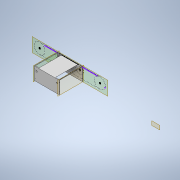
# Autodesk Inventor part: Podstawacz2
Saved by Autodesk Inventor 2022 (Build 260153000, 153)
## iProperties
Created: 2023-05-02
Part Number: Podstawacz2
Material: Ogólny
Document SubType Name: Modeling
Designer: nosal
Density: 1 g/cm^3
Appearance: Domyślna
Author: nosal
Autodesk Inventor part; units mm, degrees
sketch "Szkic1" plane through (0, 0, 0) normal (0, 0, 1) x (1, 0, 0)
  arc A0 (0, 35) -> (0, -35) centre (0, 0) ccw construction
  line L0 (0, 35) -> (390, 35) construction
  line L1 (0, -35) -> (390, -35) construction
  arc A1 (390, -35) -> (390, 35) centre (390, 0) ccw construction
  circle A2 centre (0, 0) radius 4.5
  circle A3 centre (390, 0) radius 4.5
  line L2 (130, 35) -> (130, 10) construction
  line L3 (260, 35) -> (260, 10) construction
  circle A4 centre (130, 10) radius 25 construction
  circle A5 centre (260, 10) radius 25 construction
  circle A6 centre (130, 10) radius 4.5
  circle A7 centre (260, 10) radius 4.5
  circle A8 centre (0, 0) radius 35 construction
  circle A9 centre (390, 0) radius 35 construction
  line L4 (117.8756, 33) -> (31.8551, 33)
  line L5 (375.6125, 33) -> (272.1244, 33)
  line L6 (247.8756, 33) -> (142.1244, 33)
  line L7 (31.8551, 31) -> (114.6703, 31)
  line L8 (145.3297, 31) -> (244.6703, 31)
  line L9 (275.3297, 31) -> (371.697, 31)
  arc A10 (375.6125, 33) -> (371.697, 31) centre (390, 0) ccw
  arc A11 (117.8756, 33) -> (114.6703, 31) centre (130, 10) ccw
  arc A12 (145.3297, 31) -> (142.1244, 33) centre (130, 10) ccw
  arc A13 (247.8756, 33) -> (244.6703, 31) centre (260, 10) ccw
  arc A14 (275.3297, 31) -> (272.1244, 33) centre (260, 10) ccw
  line L10 (31.8551, 14.5) -> (31.8551, 35) construction
  line L11 (31.8551, 33) -> (31.8551, 31)
  line L12 (260, 10) -> (260, 0)
  line L13 (130, 10) -> (130, 0)
  point P0 (423.5971, -9.8098)
  dimension "d94" = 50
  dimension "d0" = 70
  dimension "d1" = 390
  dimension "d2" = 390
  dimension "d3" = 70
  dimension "d4" = 9
  dimension "d5" = 9
  dimension "d10" = 25
  dimension "d11" = 25
  dimension "d12" = 9
  dimension "d13" = 9
  dimension "d14" = 130
  dimension "d15" = 260
  dimension "d24" = 2
  dimension "d25" = 2
  dimension "d26" = 2
  dimension "d27" = 1
  dimension "d95" = 2
  constraints: 28 end point, 17 point on circle, 13 centre point, 9 coincident, 6 point on line, 2 horizontal, 2 perpendicular, 2 tangent, 2 vertical, 2 vertical alignment, 1 concentric, 4 other
  measures "d0" diameter of A0
  measures "d1" distance of L0.start L0.end
  measures "d2" distance of L1.start L1.end
  measures "d3" diameter of A1
  measures "d4" diameter of A2
  measures "d5" diameter of A3
  measures "d10" distance of L2.start L2.end
  measures "d11" distance of L3.start L3.end
  measures "d12" diameter of A6
  measures "d13" diameter of A7
  measures "d14" distance between parallel lines of L3 L2
  measures "d15" distance from line of point (0, 0) L3
  measures "d24" distance between parallel lines of L4 L7
  measures "d25" distance between parallel lines of L6 L8
  measures "d26" distance between parallel lines of L5 L9
  measures "d27" radial gap between concentric circles of A9 A10
  measures "d95" distance between parallel lines of L0 L6
extrude "Wyciągnięcie proste1" add sketch "Szkic1" along normal blind 145 contours A11 L7 L11 L4 | A10 L9 A14 L5 | A13 L8 A12 L6
ref_plane "Płaszczyzna konstrukcyjna1" through (117.8756, 33, 145) normal (0, 0, 1) x (-1, 0, 0)
sketch "Szkic3" plane through (117.8756, 33, 145) normal (0, 0, 1) x (-1, 0, 0)
  circle A0 centre (117.8756, 33) radius 4.5 projected
  arc A1 (133.7659, 28.5) -> (133.7659, 37.5) centre (133.7659, 33) ccw
  arc A2 (98.6659, 37.5) -> (98.6659, 28.5) centre (98.6659, 33) ccw
  line L0 (133.7659, 28.5) -> (98.6659, 28.5)
  line L1 (98.6659, 37.5) -> (133.7659, 37.5)
  line L2 (98.6659, 18.5) -> (133.7659, 18.5)
  arc A3 (133.7659, 18.5) -> (133.7659, 47.5) centre (133.7659, 33) ccw
  line L3 (133.7659, 47.5) -> (98.6659, 47.5)
  line L4 (86.0205, 18.5) -> (86.0205, -2) construction
  line L5 (98.6659, 18.5) -> (86.0205, 18.5)
  line L6 (98.6659, 47.5) -> (86.0205, 47.5)
  line L7 (86.0205, 0) -> (86.0205, 2) projected
  line L8 (86.0205, 18.5) -> (86.0205, 0)
  line L9 (98.6659, 47.5) -> (98.6659, 81.8113)
  line L10 (98.6659, 81.8113) -> (-234.1244, 81.8113)
  line L11 (-157.4541, 2) -> (-253.8214, 2) projected
  line L12 (86.0205, 0) -> (86.0205, 2)
  line L13 (-257.7369, 0) -> (-154.2487, 0) projected
  line L14 (86.0205, 0) -> (-238.0399, 0)
  circle A4 centre (-272.1244, 33) radius 35 construction
  line L15 (-234.1244, 2) -> (-234.1244, 18.5)
  line L16 (-234.1244, 2) -> (-238.0399, 0)
  line L17 (-246.7694, 47.5) -> (-246.7694, 81.8113)
  line L18 (-246.7694, 81.8113) -> (-234.1244, 81.8113)
  line L19 (-303.9795, 47.5) -> (-409.6259, 47.5) construction
  line L20 (-234.1244, 47.5) -> (-246.7694, 47.5)
  line L21 (-234.1244, 18.5) -> (-281.8694, 18.5)
  line L22 (-246.7694, 47.5) -> (-281.8694, 47.5)
  arc A5 (-281.8694, 47.5) -> (-281.8694, 18.5) centre (-281.8694, 33) ccw
  point P0 (-238.0399, 0)
  dimension "d33" = 9
  dimension "d34" = 9
  dimension "d35" = 10
  dimension "d36" = 47.7454
  dimension "d37" = 12.6455
  dimension "d38" = 12.6455
  dimension "d39" = 12.6455
  dimension "d40" = 0
  dimension "d64" = 47.745
  dimension "d93" = 16.5
  constraints: 38 end point, 8 point on circle, 5 horizontal, 4 centre point, 3 parallel, 3 tangent, 3 vertical, 2 collinear, 2 perpendicular, 2 point on line, 4 other
  measures "d33" diameter of A1
  measures "d34" diameter of A2
  measures "d35" distance between parallel lines of L0 L2
  measures "d36" distance from line of L3.start L4
  measures "d37" distance from line of L3.end L4
  measures "d38" distance from line of L1.start L4
  measures "d39" distance from line of L2.start L4
  measures "d40" distance from line of L6.end L4
  measures "d64" distance of L15.end L21.end
  measures "d93" distance of L15.start L15.end
extrude "Wyciągnięcie proste2" add sketch "Szkic3" along normal blind 4
ref_plane "Płaszczyzna konstrukcyjna4" through (117.8756, 33, 72.5) normal (0, 0, -1) x (-1, 0, 0)
mirror "Odbij2" about plane through (117.8756, 33, 72.5) normal (0, 0, -1) of "Wyciągnięcie proste2"
extrude "Wyciągnięcie proste4" cut sketch "Szkic1" along normal mid plane 10000 contours A6 | A7
sketch "Szkic8" plane through (0, 0, 145) normal (0, 0, 1) x (1, 0, 0)
  line L0 (352, 31) -> (371.697, 31) projected
  line L1 (352, 31) -> (355.9155, 33) projected
  line L2 (352, 31) -> (355.9155, 33)
  line L3 (375.6125, 33) -> (355.9155, 33) projected
  line L4 (355.9155, 33) -> (375.6125, 33)
  arc A0 (375.6125, 33) -> (371.697, 31) centre (390, 0) ccw projected
  line L5 (375.6125, 33) -> (371.697, 31)
  line L6 (352, 14.5) -> (352, 31) projected
  line L7 (371.697, 31) -> (352, 31)
  point P0 (0, 0)
  point P1 (352, -48.8113)
  constraints: 8 end point, 3 equal length, 1 perpendicular
ref_plane "Płaszczyzna konstrukcyjna6" through (0, 0, 72.5) normal (0, 0, 1) x (1, 0, 0)
extrude "Wyciągnięcie proste5" cut sketch "Szkic8" along normal mid plane 1000 contours L1 L3 A0 L0
ref_plane "Płaszczyzna konstrukcyjna9" through (117.8756, 33, 149) normal (0, 0, 1) x (1, 0, 0)
sketch "Szkic12" plane through (117.8756, 33, 149) normal (0, 0, 1) x (1, 0, 0)
  line L0 (281.8694, -18.5) -> (234.1244, -18.5) projected
  arc A0 (281.8694, -47.5) -> (281.8694, -18.5) centre (281.8694, -33) ccw projected
  line L1 (246.7694, -47.5) -> (281.8694, -47.5) projected
  line L2 (246.7694, -81.8113) -> (246.7694, -47.5) projected
  line L3 (234.1244, -2) -> (234.1244, -81.8113) projected
  line L4 (-98.6659, -81.8113) -> (246.7694, -81.8113) projected
  point P0 (-117.8756, -33)
extrude "Wyciągnięcie proste7" cut sketch "Szkic12" against normal blind 17
extrude "Wyciągnięcie proste8" cut sketch "Szkic1" against normal blind 17 contours A3
ref_plane "Płaszczyzna konstrukcyjna10" through (117.8756, 33, 149) normal (0, 0, 1) x (1, 0, 0)
sketch "Szkic13" plane through (117.8756, 33, 149) normal (0, 0, 1) x (1, 0, 0)
  line L0 (234.1244, -81.8113) -> (234.1244, -2) projected
  line L1 (232.1244, -81.8113) -> (232.1244, -2)
  line L2 (234.1244, -2) -> (238.0399, 0) projected
  line L3 (238.0399, 0) -> (236.0399, 0)
  line L4 (238.0399, 0) -> (-86.0205, 0) projected
  line L5 (236.0399, 0) -> (232.1244, -2)
  line L6 (238.0399, 0) -> (234.1244, -2)
  line L7 (234.1244, -81.8113) -> (232.1244, -81.8113)
  line L8 (-98.6659, -81.8113) -> (246.7694, -81.8113) projected
  point P0 (-117.8756, -33)
  dimension "d70" = 2
  dimension "d71" = 2
  constraints: 10 end point, 2 parallel, 1 collinear, 1 point on line
  measures "d70" distance between parallel lines of L0 L1
  measures "d71" distance of L2.end L3.end
extrude "Wyciągnięcie proste9" add sketch "Szkic13" along normal blind 17
ref_plane "Płaszczyzna konstrukcyjna11" through (117.8756, 33, 166) normal (0, 0, 1) x (1, 0, 0)
sketch "Szkic14" plane through (117.8756, 33, 166) normal (0, 0, 1) x (1, 0, 0)
  line L0 (232.1244, -81.8113) -> (234.1244, -81.8113) projected
  line L1 (-98.6659, -81.8113) -> (246.7694, -81.8113) projected
  line L2 (232.1244, -81.8113) -> (246.7694, -81.8113)
  line L3 (246.7694, -81.8113) -> (246.7694, -47.5) projected
  line L4 (246.7694, -81.8113) -> (246.7694, -47.5)
  line L5 (246.7694, -47.5) -> (281.8694, -47.5) projected
  line L6 (246.7694, -47.5) -> (281.8694, -47.5)
  line L7 (281.8694, -18.5) -> (234.1244, -18.5) projected
  line L8 (234.1244, -81.8113) -> (234.1244, -2) projected
  arc A0 (281.8694, -47.5) -> (281.8694, -18.5) centre (281.8694, -33) ccw projected
  circle A1 centre (272.1244, -33) radius 4.5 projected
  line L9 (232.1244, -2) -> (232.1244, -81.8113) projected
  line L10 (236.0399, 0) -> (232.1244, -2) projected
  line L11 (238.0399, 0) -> (236.0399, 0) projected
  line L12 (234.1244, -2) -> (238.0399, 0) projected
  point P0 (-117.8756, -33)
  constraints: 6 end point, 2 perpendicular, 1 collinear
extrude "Wyciągnięcie proste10" add sketch "Szkic14" along normal blind 4
ref_plane "Płaszczyzna konstrukcyjna12" through (364.645, -48.8113, -4) normal (0, 0, -1) x (-1, 0, 0)
sketch "Szkic15" plane through (364.645, -48.8113, -4) normal (0, 0, -1) x (-1, 0, 0)
  line L0 (332.7899, 63.3113) -> (322.7899, 63.3113)
  line L1 (322.7899, 63.3113) -> (322.7899, 34.3113)
  line L2 (322.7899, 34.3113) -> (332.7899, 34.3113)
  line L3 (332.7899, 34.3113) -> (332.7899, 63.3113)
  point P0 (364.645, 48.8113)
  dimension "d78" = 10
  constraints: 8 end point, 2 parallel, 1 horizontal, 1 perpendicular
  measures "d78" distance of L2.end L1.end
extrude "Wyciągnięcie proste11" add sketch "Szkic15" along normal blind 14.44
ref_plane "Płaszczyzna konstrukcyjna13" through (117.8756, 33, 149) normal (0, 0, 1) x (1, 0, 0)
sketch "Szkic16" plane through (117.8756, 33, 149) normal (0, 0, 1) x (1, 0, 0)
  line L0 (-86.0205, -18.5) -> (-133.7659, -18.5) projected
  line L1 (-86.0205, -47.5) -> (-76.0205, -47.5) projected
  line L2 (-86.0205, -18.5) -> (-76.0205, -18.5)
  line L3 (-76.0205, -18.5) -> (-76.0205, -47.5)
  line L4 (-76.0205, -47.5) -> (-86.0205, -47.5)
  line L5 (-86.0205, -47.5) -> (-86.0205, -18.5)
  point P0 (-117.8756, -33)
  point P1 (-86.0205, -47.5)
  dimension "d82" = 10
  constraints: 8 end point, 2 parallel, 1 horizontal, 1 perpendicular
  measures "d82" distance of L1.end L4.end
extrude "Wyciągnięcie proste12" add sketch "Szkic16" along normal blind 14.44
ref_plane "Płaszczyzna konstrukcyjna14" through (31.8551, -14.5, -4) normal (-1, 0, 0) x (0, 0, 1)
sketch "Szkic17" plane through (31.8551, -14.5, -4) normal (-1, 0, 0) x (0, 0, 1)
  line L0 (4, 0) -> (4, 29) projected
  line L1 (4, 19) -> (-14.44, 19)
  line L2 (-14.44, 29) -> (-14.44, 0) projected
  line L3 (4, 10) -> (0, 10) projected
  line L4 (4, 10) -> (-12.44, 10)
  line L5 (4, 18.5) -> (-12.44, 18.5)
  line L6 (-12.44, 18.5) -> (-4.44, 18.5)
  line L7 (-4.44, 18.5) -> (-4.44, 10.5)
  line L8 (-4.44, 10.5) -> (-12.44, 10.5)
  line L9 (-12.44, 10.5) -> (-12.44, 18.5)
  circle A0 centre (-8.44, 14.5) radius 2.5
  point P0 (4, 14.5)
  dimension "d86" = 9
  dimension "d87" = 0.5
  dimension "d88" = 8
  dimension "d89" = 8
  dimension "d90" = 5
  constraints: 14 end point, 4 parallel, 3 horizontal, 2 point on line, 1 centre point, 1 perpendicular
  measures "d86" distance between parallel lines of L4 L1
  measures "d87" distance between parallel lines of L1 L5
  measures "d88" distance of L7.end L8.end
  measures "d89" distance of L6.end L7.end
  measures "d90" diameter of A0
extrude "Wyciągnięcie proste13" cut sketch "Szkic17" against normal through all contours A0
mirror "Odbij3" about plane through (117.8756, 33, 72.5) normal (0, 0, -1) of "Wyciągnięcie proste13"
ref_plane "Płaszczyzna konstrukcyjna15" through (364.645, -48.8113, -4) normal (0, 0, -1) x (-1, 0, 0)
sketch "Szkic19" plane through (364.645, -48.8113, -4) normal (0, 0, -1) x (-1, 0, 0)
  circle A0 centre (234.645, 58.8113) radius 4.5 projected
  line L0 (234.645, 58.8113) -> (249.645, 58.8113)
  circle A1 centre (104.645, 58.8113) radius 4.5 projected
  line L1 (104.645, 58.8113) -> (89.645, 58.8113)
  line L2 (89.645, 101.2973) -> (-85.4155, 101.2973)
  line L3 (-85.4155, 101.2973) -> (-85.4155, -16.8317)
  line L4 (-85.4155, -16.8317) -> (89.645, -16.8317)
  line L5 (89.645, -16.8317) -> (89.645, 101.2973)
  line L6 (249.645, 101.2973) -> (438.4161, 101.2973)
  line L7 (438.4161, 101.2973) -> (438.4161, -28.5413)
  line L8 (438.4161, -28.5413) -> (249.645, -28.5413)
  line L9 (249.645, -28.5413) -> (249.645, 101.2973)
  point P0 (364.645, 48.8113)
  dimension "d99" = 15
  dimension "d100" = 15
  constraints: 20 end point, 4 horizontal, 4 parallel, 2 perpendicular
  measures "d99" distance of L0.start L0.end
  measures "d100" distance of L1.start L1.end
extrude "Wyciągnięcie proste14" cut sketch "Szkic19" along normal mid plane 682 contours L9 L6 L7 L8 | L5 L4 L3 L2
ref_plane "Płaszczyzna konstrukcyjna17" through (115, -48.8113, 149) normal (-1, 0, 0) x (0, 0, 1)
sketch "Szkic21" plane through (115, -48.8113, 149) normal (-1, 0, 0) x (0, 0, 1)
  line L0 (-149, 0) -> (-153, 0) projected
  line L1 (-151, 0) -> (-151, 15)
  line L2 (0, 0) -> (-4, 0) projected
  line L3 (-2, 0) -> (-2, 15)
  line L4 (0, 81.8113) -> (0, 0) projected
  line L5 (0, 81.8113) -> (-153, 81.8113) projected
  line L6 (-2, 81.8113) -> (-2, 66.8113)
  line L7 (-151, 81.8113) -> (-151, 66.8113)
  circle A0 centre (-151, 66.8113) radius 1
  circle A1 centre (-2, 66.8113) radius 1
  circle A2 centre (-2, 15) radius 1
  circle A3 centre (-151, 15) radius 1
  point P0 (-149, 48.8113)
  dimension "d112" = 15
  dimension "d113" = 15
  dimension "d114" = 15
  dimension "d115" = 2
  dimension "d116" = 2
  dimension "d117" = 2
  dimension "d118" = 2
  constraints: 8 end point, 4 centre point, 4 coincident, 2 midpoint, 2 point on line, 2 vertical, 1 parallel, 1 perpendicular
  measures "d112" distance of L6.start L6.end
  measures "d113" distance of L3.start L3.end
  measures "d114" distance of L1.start L1.end
  measures "d115" diameter of A0
  measures "d116" diameter of A1
  measures "d117" diameter of A2
  measures "d118" diameter of A3
extrude "Wyciągnięcie proste15" cut sketch "Szkic21" against normal blind 7
ref_plane "Płaszczyzna konstrukcyjna18" through (275, -48.8113, -4) normal (1, 0, 0) x (0, 0, -1)
sketch "Szkic22" plane through (275, -48.8113, -4) normal (1, 0, 0) x (0, 0, -1)
  circle A0 centre (-151, 66.8113) radius 1 projected
  circle A1 centre (-151, 15) radius 1 projected
  circle A2 centre (-2, 66.8113) radius 1 projected
  line L0 (-4, 80.0481) -> (-4, 0) projected
  circle A3 centre (-2, 15) radius 1 projected
  point P0 (-4, 48.8113)
extrude "Wyciągnięcie proste16" cut sketch "Szkic22" against normal blind 7
ref_plane "Płaszczyzna konstrukcyjna5" through (117.8756, 33, 72.5) normal (0, 0, -1) x (-1, 0, 0)
